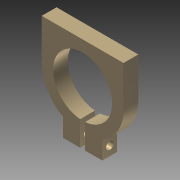
# Autodesk Inventor part: Router mount
Saved by Autodesk Inventor 2012 (Build 160160000, 160)
## iProperties
Created: 2013-05-09
Part Number: Router mount
Material: Default
Document SubType Name: Modeling
Designer: Fabian
Density: 1 g/cm^3
Author: Fabian
Autodesk Inventor part; units mm, degrees
ref_plane "YZ Plane" through (0, 0, 0) normal (1, 0, 0) x (0, 1, 0)
ref_plane "XZ Plane" through (0, 0, 0) normal (0, 1, 0) x (-1, 0, 0)
ref_plane "XY Plane" through (0, 0, 0) normal (0, 0, 1) x (1, 0, 0)
sketch "Sketch1" plane through (0, 0, 0) normal (0, 0, 1) x (1, 0, 0)
  line L0 (-72.2389, 37.814) -> (33.1711, 37.814)
  line L1 (33.1711, 37.814) -> (33.1711, 28.0212)
  line L2 (33.1711, 28.0212) -> (-72.2389, 28.0212)
  line L3 (-72.2389, 28.0212) -> (-72.2389, 37.814)
  circle A0 centre (-19.5339, -14.891) radius 38.1
  circle A1 centre (-19.5339, -14.891) radius 52.705
  line L4 (-72.2389, -14.891) -> (-72.2389, 28.0212)
  line L5 (33.1711, 28.0212) -> (33.1711, -14.891)
  line L6 (-44.9339, -61.0717) -> (-44.9339, -84.741)
  line L7 (-44.9339, -84.741) -> (5.8661, -84.741)
  line L8 (5.8661, -84.741) -> (5.8661, -61.0717)
  line L9 (-22.7089, -52.8585) -> (-22.7089, -84.741)
  line L10 (-16.3589, -84.741) -> (-16.3589, -52.8585)
  point P0 (0, 0)
  dimension "d0" = 105.41
  dimension "d1" = 105.41
  dimension "d2" = 76.2
  dimension "d3" = 52.705
  dimension "d4" = 25.4
  dimension "d5" = 25.4
  dimension "d6" = 69.85
  dimension "d7" = 22.225
  dimension "d8" = 22.225
  constraints: 22 end point, 6 point on circle, 5 parallel, 4 perpendicular, 2 centre point, 2 point on line, 2 tangent, 1 coincident, 1 horizontal
  measures "d0" distance of L0.start L0.end
  measures "d1" diameter of A1
  measures "d2" diameter of A0
  measures "d3" distance from line of L0 A0.centre
  measures "d4" distance from line of L6 A0.centre
  measures "d5" distance from line of L8 A0.centre
  measures "d6" distance from line of A1.centre L7
  measures "d7" distance between parallel lines of L6 L9
  measures "d8" distance between parallel lines of L8 L10
extrude "Extrusion1" add sketch "Sketch1" along normal blind 19.05 contours L0 A1 L2 L3 | L0 L1 L2 A1 | A1 L2 | A1 L10 A0 L9 L2 | A1 L9 L7 L6 | L8 L7 L10 A1
sketch "Sketch2" plane through (0, 0, 19.05) normal (0, 0, 1) x (1, 0, 0)
  line L0 (-50.1339, 28.0212) -> (-72.2389, 28.0212) projected
  arc A0 (-50.1339, 28.0212) -> (-44.9339, -61.0717) centre (-19.5339, -14.891) ccw projected
  arc A1 (5.8661, -61.0717) -> (11.0661, 28.0212) centre (-19.5339, -14.891) ccw projected
  line L1 (33.1711, 28.0212) -> (11.0661, 28.0212) projected
  line L2 (33.1711, 37.814) -> (33.1711, 28.0212) projected
  line L3 (-72.2389, 28.0212) -> (-72.2389, -14.891)
  line L4 (33.1711, 28.0212) -> (33.1711, -14.891)
  point P0 (0, 0)
  constraints: 4 end point, 2 point on circle, 1 parallel, 1 tangent
extrude "Extrusion2" add sketch "Sketch2" against normal blind 19.05
sketch "Sketch3" plane through (5.8661, -84.741, 0) normal (1, 0, 0) x (0, 0, -1)
  point P0 (0, 84.741)
  point P1 (-9.525, 11.8347)
hole "Hole1" at (5.8661, -72.9064, 9.525) direction (-1, 0, 0) diameter 9.525 end through all
body "Solid1"
